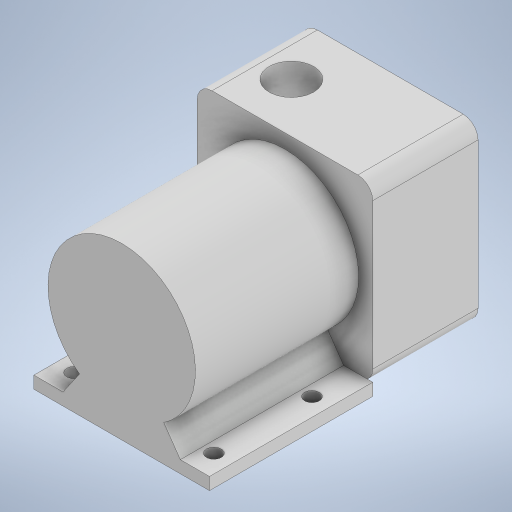
# Autodesk Inventor part: Water_pump
Saved by Autodesk Inventor 2023 (Build 270158000, 158)
## iProperties
Created: 2023-08-19
Part Number: Water_pump
Material: Generic
Document SubType Name: Modeling
Designer: plebbb
Density: 1 g/cm^3
Appearance: Default
Author: plebbb
Autodesk Inventor part; units mm, degrees
ref_plane "YZ Plane" through (0, 0, 0) normal (1, 0, 0) x (0, 1, 0)
ref_plane "XZ Plane" through (0, 0, 0) normal (0, 1, 0) x (-1, 0, 0)
ref_plane "XY Plane" through (0, 0, 0) normal (0, 0, 1) x (1, 0, 0)
sketch "Sketch1" plane through (0, 0, 0) normal (0, 0, 1) x (1, 0, 0)
  line L0 (0, 0) -> (50, 0)
  line L1 (50, 0) -> (50, 50)
  line L2 (50, 50) -> (0, 50)
  line L3 (0, 50) -> (0, 0)
  line L4 (5.3353, 5.3353) -> (44.6647, 5.3353) construction
  line L5 (44.6647, 5.3353) -> (44.6647, 44.6647) construction
  line L6 (44.6647, 44.6647) -> (5.3353, 44.6647) construction
  line L7 (5.3353, 44.6647) -> (5.3353, 5.3353) construction
  line L8 (25, 44.6647) -> (25, 50) construction
  line L9 (44.6647, 25) -> (50, 25) construction
  dimension "d0" = 50
  constraints: 20 end point, 4 midpoint, 4 parallel, 4 perpendicular, 3 horizontal, 1 vertical
  measures "d0" distance of L1.end L2.end
extrude "Extrusion1" add sketch "Sketch1" along normal blind 30
sketch "Sketch2" plane through (0, 0, 30) normal (0, 0, 1) x (1, 0, 0)
  line L0 (0, -2.5) -> (50, -2.5)
  line L1 (50, -2.5) -> (50, 1)
  line L2 (50, 1) -> (0, 1)
  line L3 (0, 1) -> (0, -2.5)
  circle A0 centre (25, 25) radius 21
  line L4 (50, 50) -> (0, 50) construction
  line L5 (50, 0) -> (50, 50) construction
  line L6 (25, 25) -> (25, 50) construction
  line L7 (25, 25) -> (50, 25) construction
  line L8 (13, 7.7663) -> (37, 7.7663)
  line L9 (8.2885, 1) -> (25, 25)
  line L10 (25, 25) -> (41.7115, 1)
  point P0 (0, 0)
  point P1 (0, -0.75)
  point P2 (50, -0.75)
  dimension "d3" = 2.5
  dimension "d4" = 3.5
  dimension "d5" = 42
  dimension "d6" = 24
  constraints: 18 end point, 4 midpoint, 4 point on line, 2 horizontal, 2 parallel, 2 perpendicular, 2 point on circle, 2 vertical alignment, 1 centre point, 1 vertical
  measures "d3" distance from line of point (0, 0) L0
  measures "d4" distance of L2.end L0.start
  measures "d5" diameter of A0
  measures "d6" distance of L8.start L8.end
extrude "Extrusion2" add sketch "Sketch2" along normal blind 46.5
sketch "Sketch3" plane through (0, -2.5, 30) normal (0, -1, 0) x (1, 0, 0)
  line L0 (44.8967, 40.15) -> (5.1033, 40.15) construction
  line L1 (5.1033, 40.15) -> (5.1033, 12.21) construction
  line L2 (5.1033, 12.21) -> (44.8967, 12.21) construction
  line L3 (44.8967, 12.21) -> (44.8967, 40.15) construction
  line L4 (0, 46.5) -> (50, 46.5) construction
  line L5 (25, 40.15) -> (25, 46.5) construction
  circle A0 centre (44.8967, 40.15) radius 2.1167
  circle A1 centre (44.8967, 12.21) radius 2.1167
  circle A2 centre (5.1033, 40.15) radius 2.1167
  circle A3 centre (5.1033, 12.21) radius 2.1167
  point P0 (0, -30)
  dimension "d9" = 27.94
  dimension "d10" = 6.35
  dimension "d11" = 39.7933
  dimension "d12" = 4.2333
  constraints: 10 end point, 4 centre point, 4 coincident, 3 equal radius, 2 midpoint, 2 parallel, 1 horizontal, 1 perpendicular, 1 vertical
  measures "d9" distance of L2.end L0.start
  measures "d10" distance between parallel lines of L4 L0
  measures "d11" distance of L0.start L0.end
  measures "d12" diameter of A0
extrude "Extrusion3" cut sketch "Sketch3" against normal up to surface (3.5 mm away)
sketch "Sketch4" plane through (0, 0, 0) normal (0, 0, -1) x (-1, 0, 0)
  circle A0 centre (-25, 25) radius 6.35
  line L0 (-50, 50) -> (0, 50) construction
  line L1 (0, 50) -> (0, 0) construction
  point P0 (-25, 50)
  point P1 (0, 25)
  dimension "d15" = 12.7
  constraints: 2 midpoint, 1 centre point, 1 horizontal alignment, 1 vertical alignment
  measures "d15" diameter of A0
extrude "Extrusion4" cut sketch "Sketch4" against normal blind 10
sketch "Sketch5" plane through (0, 50, 0) normal (0, 1, 0) x (1, 0, 0)
  circle A0 centre (12.7, -15.875) radius 6.35
  point P0 (0, 0)
  dimension "d18" = 12.7
  dimension "d19" = 12.7
  dimension "d20" = 15.875
  constraints: 1 centre point
  measures "d18" diameter of A0
  measures "d19" horizontal distance of point (0, 0) A0.centre
  measures "d20" vertical distance of point (0, 0) A0.centre
extrude "Extrusion5" cut sketch "Sketch5" against normal blind 10
fillet "Fillet1" radius 4.2333 4 edges at (50, 50, 15) (0, 50, 15) (0, 0, 15) (50, 0, 15)
body "Solid1"
